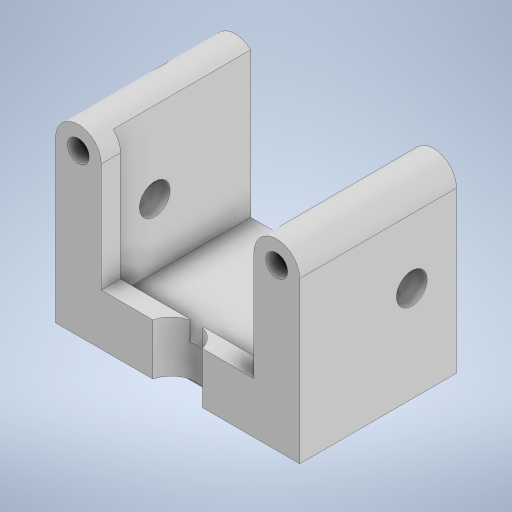
# Autodesk Inventor part: SolenoidBracket
Saved by Autodesk Inventor 2023 (Build 270158000, 158)
## iProperties
Created: 2020-02-19
Part Number: SolenoidBracket
Material: Generic
Document SubType Name: Modeling
Designer: Owner
Density: 1 g/cm^3
Appearance: Default
Author: Owner
Autodesk Inventor part; units mm, degrees
note: some values were not read from the file. Chosen so that the rebuilt part matches the saved one: direction of "Hole4"; direction of "Hole5".
ref_plane "YZ Plane" through (0, 0, 0) normal (1, 0, 0) x (0, 1, 0)
ref_plane "XZ Plane" through (0, 0, 0) normal (0, 1, 0) x (-1, 0, 0)
ref_plane "XY Plane" through (0, 0, 0) normal (0, 0, 1) x (1, 0, 0)
sketch "Sketch1" plane through (0, 0, 0) normal (0, 0, 1) x (1, 0, 0)
  line L0 (-13.075, 0) -> (13.075, 0)
  line L1 (13.075, 0) -> (13.075, 22.6856)
  line L2 (-13.075, 22.6856) -> (-13.075, 0)
  line L3 (-19.075, -5) -> (11.925, -5)
  line L4 (19.075, -5) -> (19.075, 20.0588)
  line L5 (-19.075, 20.0588) -> (-19.075, -5)
  circle A0 centre (-15.5, 20.0588) radius 1.5
  circle A1 centre (15.5, 20.0588) radius 1.5
  arc A2 (19.075, 20.0588) -> (13.075, 22.6856) centre (15.5, 20.0588) ccw
  arc A3 (-13.075, 22.6856) -> (-19.075, 20.0588) centre (-15.5, 20.0588) ccw
  line L6 (11.925, -5) -> (19.075, -5)
  point P0 (0, 0)
  dimension "d8" = 5
  dimension "d10" = 6
  dimension "d12" = 31
  dimension "d14" = 3
  dimension "d15" = 3
  dimension "d17" = 26.15
  dimension "d18" = 13.075
  dimension "d19" = 15.5
  constraints: 14 end point, 4 centre point, 4 point on circle, 3 horizontal, 2 coincident, 2 horizontal alignment, 2 parallel, 2 perpendicular, 2 tangent, 1 midpoint
  measures "d8" distance between parallel lines of L3 L0
  measures "d10" distance between parallel lines of L2 L5
  measures "d12" distance of A1.centre A0.centre
  measures "d14" diameter of A1
  measures "d15" diameter of A0
  measures "d17" distance of L0.start L0.end
  measures "d18" distance from line of L1 point (0, 0)
  measures "d19" horizontal distance of point (0, 0) A1.centre
extrude "Extrusion1" add sketch "Sketch1" along normal blind 20.5 contours L0 L1 A2 L4 L6 L3 L5 A3 L2 | A0 | A1
sketch "Sketch4" plane through (0, 0, 20.5) normal (0, 0, 1) x (1, 0, 0)
  arc A0 (-11.925, 20.0588) -> (-19.075, 20.0588) centre (-15.5, 20.0588) ccw
  arc A1 (19.075, 20.0588) -> (11.925, 20.0588) centre (15.5, 20.0588) ccw
  arc A2 (19.075, 20.0588) -> (13.075, 22.6856) centre (15.5, 20.0588) ccw projected
  arc A3 (-13.075, 22.6856) -> (-19.075, 20.0588) centre (-15.5, 20.0588) ccw projected
  line L0 (-19.075, -5) -> (19.075, -5) projected
  line L1 (19.075, -5) -> (19.075, 20.0588) projected
  arc A4 (19.075, 20.0588) -> (13.075, 22.6856) centre (15.5, 20.0588) ccw projected
  line L2 (13.075, 22.6856) -> (13.075, 0) projected
  line L3 (13.075, 0) -> (-13.075, 0) projected
  line L4 (-13.075, 0) -> (-13.075, 22.6856) projected
  arc A5 (-13.075, 22.6856) -> (-19.075, 20.0588) centre (-15.5, 20.0588) ccw projected
  line L5 (-19.075, 20.0588) -> (-19.075, -5) projected
  line L6 (-11.925, 20.0588) -> (-11.925, 3)
  line L7 (-11.925, 3) -> (11.925, 3)
  line L8 (11.925, 3) -> (11.925, 20.0588)
  point P0 (0, 0)
  point P1 (13.075, 22.6856)
  point P2 (13.075, 22.6856)
  dimension "d37" = 3
  constraints: 8 end point, 4 point on circle, 3 tangent, 2 centre point, 2 concentric, 2 vertical, 1 perpendicular
  measures "d37" distance between parallel lines of L3 L7
extrude "Extrusion3" add sketch "Sketch4" along normal blind 3
sketch "Sketch5" plane through (0, 0, 23.5) normal (0, 0, 1) x (1, 0, 0)
  arc A0 (-13.075, 22.6856) -> (-19.075, 20.0588) centre (-15.5, 20.0588) ccw projected
  arc A1 (19.075, 20.0588) -> (13.075, 22.6856) centre (15.5, 20.0588) ccw projected
  point P0 (0, 0)
  constraints: 2 coincident
hole "Hole2" at (-15.5, 20.0588, 23.5) at (15.5, 20.0588, 23.5) direction (0, 0, -1) diameter 3.4 end through all clearance for "Socket Head Cap Screw" size "M3" standard "Ansi Metric M Profile"
sketch "Sketch8" plane through (-13.075, 0, 0) normal (0, 1, 0) x (1, 0, 0)
  circle A0 centre (13.075, -24.5) radius 4
  line L0 (25, -23.5) -> (1.15, -23.5) projected
  point P0 (13.075, 0)
  dimension "d62" = 8
  dimension "d63" = 1
  constraints: 1 centre point
  measures "d62" diameter of A0
  measures "d63" distance from line of L0 A0.centre
extrude "Extrusion5" cut sketch "Sketch8" against normal through all both and the other way through all
sketch "Sketch9" plane through (-13.075, 0, 0) normal (0, 1, 0) x (1, 0, 0)
  line L0 (12.075, -28.8924) -> (14.075, -28.8924)
  line L1 (14.075, -28.8924) -> (14.075, -18.1034)
  line L2 (14.075, -18.1034) -> (12.075, -18.1034)
  line L3 (12.075, -18.1034) -> (12.075, -28.8924)
  line L4 (12.075, -28.8924) -> (14.075, -18.1034) construction
  line L5 (14.075, -28.8924) -> (12.075, -18.1034) construction
  point P0 (13.075, 0)
  point P1 (13.075, -23.4979)
  dimension "d66" = 2
  constraints: 12 end point, 2 midpoint, 2 parallel, 1 horizontal, 1 perpendicular
  measures "d66" distance of L2.end L1.end
extrude "Extrusion6" cut sketch "Sketch9" along normal blind 10
sketch "Sketch10" plane through (19.075, -5, 0) normal (1, 0, 0) x (0, 0, -1)
  circle A0 centre (-6, 14.9996) radius 2
  line L0 (0, 0) -> (-23.5, 0) projected
  line L1 (0, 0) -> (0, 25.0588) projected
  line L2 (0, 27.6856) -> (-20.5, 27.6856) projected
  point P0 (0, 5)
  dimension "d70" = 6
  dimension "d71" = 4
  dimension "d88" = 12.686
  constraints: 1 centre point
  measures "d70" distance from line of L1 A0.centre
  measures "d71" diameter of A0
  measures "d88" distance from line of A0.centre L2
hole "Hole4" at (19.075, 9.9996, 6) direction (-1, 0, 0) diameter 4.8 depth 6 clearance for "Socket Head Cap Screw" size "M4" standard "Ansi Metric M Profile"
sketch "Sketch11" plane through (-19.075, -5, 0) normal (-1, 0, 0) x (0, 0, 1)
  circle A0 centre (14, 14.9996) radius 3.2686
  line L0 (0, 0) -> (23.5, 0) projected
  circle A1 centre (6, 14.9996) radius 2.4 projected
  line L1 (0, 27.6856) -> (20.5, 27.6856) projected
  point P0 (0, 5)
  point P1 (10.9595, 8.3093)
  dimension "d80" = 8
  dimension "d89" = 12.686
  constraints: 1 centre point
  measures "d80" distance of A0.centre A1.centre
  measures "d89" distance from line of L1 A0.centre
hole "Hole5" at (-19.075, 9.9996, 14) direction (1, 0, 0) diameter 4.8 depth 6 clearance for "Socket Head Cap Screw" size "M4" standard "Ansi Metric M Profile"
sketch "Sketch12" plane through (-19.075, -5, 0) normal (0, -1, 0) x (1, 0, 0)
  line L0 (38.15, 0) -> (38.15, 23.5) projected
  circle A0 centre (0, 8) radius 1.5
  line L1 (0, 0) -> (0, 23.5) projected
  line L2 (0, 0) -> (38.15, 0) projected
  point P0 (19.075, 0)
  dimension "d93" = 3
  dimension "d94" = 8
  constraints: 1 centre point, 1 point on line
  measures "d93" diameter of A0
  measures "d94" distance from line of L2 A0.centre
extrude "Extrusion7" cut sketch "Sketch12" against normal through all
sketch "Sketch13" plane through (0, 0, 0) normal (0, 0, -1) x (-1, 0, 0)
  circle A0 centre (15.5, 20.0588) radius 1.7 projected
  circle A1 centre (-15.5, 20.0588) radius 1.7 projected
  line L0 (19.075, 20.0588) -> (19.075, -5) projected
  arc A2 (19.075, 20.0588) -> (13.075, 22.6856) centre (15.5, 20.0588) ccw projected
  line L1 (13.075, 0) -> (13.075, 22.6856) projected
  line L2 (-13.075, 0) -> (13.075, 0) projected
  line L3 (-13.075, 22.6856) -> (-13.075, 0) projected
  arc A3 (-13.075, 22.6856) -> (-19.075, 20.0588) centre (-15.5, 20.0588) ccw projected
  line L4 (-19.075, -5) -> (-19.075, 20.0588) projected
  line L5 (19.075, -5) -> (-19.075, -5) projected
  line L6 (-4.8329, -8.7412) -> (5.1671, -8.7412) projected
  line L7 (-10, -1.2588) -> (10, -1.2588)
  line L8 (10, -1.2588) -> (10, -8.7412)
  line L9 (10, -8.7412) -> (-10, -8.7412)
  line L10 (-10, -8.7412) -> (-10, -1.2588)
  line L11 (19.075, -5) -> (-19.075, -5) projected
  line L12 (-10, -1.2588) -> (10, -8.7412) construction
  line L13 (10, -1.2588) -> (-10, -8.7412) construction
  point P0 (0, 0)
  point P1 (0, -5)
  point P2 (-10, -5)
  point P3 (10, -5)
  dimension "d95" = 20
  constraints: 12 end point, 3 midpoint, 2 parallel, 1 horizontal, 1 perpendicular, 1 point on line
  measures "d95" distance of L7.start L7.end
extrude "Extrusion8" add sketch "Sketch13" against normal blind 17 contours L8 L9 L6 L10 L5
move faces "Move1" translate (0, 0, -1) faces at (-17.075, 5.0196, 0)
body "Solid1"
